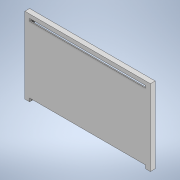
# Autodesk Inventor part: placa
Saved by Autodesk Inventor 2022 (Build 260153000, 153)
## iProperties
Created: 2022-03-04
Part Number: placa
Material: Generic
Document SubType Name: Modeling
Designer: Oana
Density: 1 g/cm^3
Appearance: Default
Author: Oana
Autodesk Inventor part; units mm, degrees
ref_plane "YZ Plane" through (0, 0, 0) normal (1, 0, 0) x (0, 1, 0)
ref_plane "XZ Plane" through (0, 0, 0) normal (0, 1, 0) x (-1, 0, 0)
ref_plane "XY Plane" through (0, 0, 0) normal (0, 0, 1) x (1, 0, 0)
sketch "Sketch1" plane through (0, 0, 0) normal (0, 0, 1) x (1, 0, 0)
  line L0 (-74.2195, 17.5033) -> (-69.2195, 17.5033)
  line L1 (-69.2195, 17.5033) -> (-69.2195, -62.4967)
  line L2 (-69.2195, -62.4967) -> (-74.2195, -62.4967)
  line L3 (-74.2195, -62.4967) -> (-74.2195, 17.5033)
  line L4 (-69.2195, 17.5033) -> (52.7805, 17.5033)
  line L5 (52.7805, 17.5033) -> (52.7805, 13.4578)
  line L6 (52.7805, 13.4578) -> (-69.2195, 13.4578)
  line L7 (-69.2195, 13.4578) -> (-69.2195, 17.5033)
  line L8 (52.7805, 17.5033) -> (57.7805, 17.5033)
  line L9 (57.7805, 17.5033) -> (57.7805, -62.4967)
  line L10 (57.7805, -62.4967) -> (52.7805, -62.4967)
  line L11 (52.7805, -62.4967) -> (52.7805, 17.5033)
  point P0 (0, 0)
  point P1 (-69.2195, 13.4578)
  dimension "d0" = 5
  dimension "d1" = 80
  dimension "d2" = 122
  constraints: 24 end point, 6 parallel, 3 horizontal, 3 perpendicular, 1 collinear, 1 point on line
  measures "d0" distance of L0.start L0.end
  measures "d1" distance of L2.end L0.start
  measures "d2" distance of L0.end L4.end
extrude "Extrusion1" add sketch "Sketch1" along normal blind 5
sketch "Sketch2" plane through (-69.2195, -62.4967, 0) normal (1, 0, 0) x (0, 0, -1)
  point P0 (0, 62.4967)
sketch "Sketch3" plane through (-69.2195, -62.4967, 0) normal (1, 0, 0) x (0, 0, -1)
  point P0 (0, 62.4967)
sketch "Sketch4" plane through (-69.2195, -62.4967, 0) normal (1, 0, 0) x (0, 0, -1)
  line L0 (-5, 73.4545) -> (-4, 73.4545)
  line L1 (-4, 73.4545) -> (-4, 3.4545)
  line L2 (-4, 3.4545) -> (-5, 3.4545)
  line L3 (-5, 3.4545) -> (-5, 73.4545)
  line L4 (-5, 0) -> (-5, 75.9545) projected
  line L5 (0, 75.9545) -> (-5, 75.9545) projected
  line L6 (0, 0) -> (-5, 0) projected
  point P0 (0, 62.4967)
  point P1 (-5, 38.4545)
  dimension "d5" = 1
  dimension "d6" = 70
  dimension "d7" = 2.5
  dimension "d8" = 3.4545
  constraints: 8 end point, 2 parallel, 1 horizontal, 1 midpoint, 1 perpendicular, 1 point on line
  measures "d5" distance of L1.end L2.end
  measures "d6" distance of L0.end L1.end
  measures "d7" distance between parallel lines of L5 L0
  measures "d8" distance between parallel lines of L6 L2
extrude "Extrusion2" add sketch "Sketch4" along normal up to surface (122 mm away)
body "Solid1"
